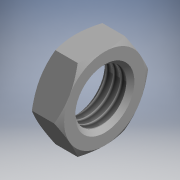
# Autodesk Inventor part: SNJ-010C
Saved by Autodesk Inventor 2017.3 (Build 213256000, 256)
## iProperties
Part Number: SNJ-010C
Material: Generic
Catalog Web Link: www.cadenas.de
Description: CJ2-Z_SNJ-Mounting Nut
Vendor: SMC
Document SubType Name: Modeling
Designer: partserver
Manufacturer: SMC
Mass: 0.259253 g
Surface Area: 3.5092 cm^2
Volume: 0.259253 cm^3
Density: 1 g/cm^3
Appearance: PSOLRGB-191-191-191
Category: PARTsolutions
Company: SMC
Title: SNJ-010C
Author: Cadenas PARTsolutions
Comments: Mounting Nut
PSOL_IDENT_0: {$CADENAS_DATA\23d-libs\smc_jp\actuator\standard_air_cylinder\cj2\accessories\cj2_z_snj.prj},159 {VT
PSOL_IDENT_1: YP=3D},{NB=SNJ-010C},{LINA=SNJ-010C},{NN=CJ2-Z_SNJ},{DATE=04.02.2022 06:57:30},{GEOMDATE=12.05.2020
PSOL_IDENT_2: 08:15:39},{VERSION=},{LINEID=90},{WBVAR=},{WBNUMERIC=}  {NB=SNJ-010C},{LINA=SNJ-010C},{KT=DUMMY},{MO
PSOL_IDENT_3: DEL=SNJ-010C},{BORE=10},{B1=11},{C1=12.7},{D=M8x1.0},{D1=8},{D2=1},{H1=4},{ORDER=SNJ-010C}
NB: SNJ-010C
NN: CJ2-Z_SNJ
NT: Mounting Nut
NBSYN: $MODEL.
LINA: SNJ-010C
CATALOG: SMC (JP
MODEL: SNJ-010C
BORE: 10
B1: 11
C1: 12.7
D: M8x1.0
H1: 4
SUPPLIER: SMC
ARTICLENO: SNJ-010C
BOMINFO: SNJ-010C
CREATOR: CADENAS GmbH
Autodesk Inventor part; units mm, degrees
sketch "B" plane through (0, 0, 0) normal (1, 0, 0) x (0, 1, 0)
  line L0 (-3.1754, 5.5) -> (-6.3509, 0)
  line L1 (-6.3509, 0) -> (-3.1754, -5.5)
  line L2 (-3.1754, -5.5) -> (3.1754, -5.5)
  line L3 (3.1754, -5.5) -> (6.3509, 0)
  line L4 (6.3509, 0) -> (3.1754, 5.5)
  line L5 (3.1754, 5.5) -> (-3.1754, 5.5)
  constraints: 12 end point
extrude "Extrusion1" add sketch "B" along normal mid plane 4
sketch "Sketch_2" plane through (0, 0, 0) normal (0, 0, 1) x (1, 0, 0)
  line L0 (2, 0) -> (-2, 0)
  line L1 (-2, 0) -> (-2, 4)
  line L2 (-2, 4) -> (-1.4585, 3.4585)
  line L3 (-1.4585, 3.4585) -> (1.4585, 3.4585)
  line L4 (1.4585, 3.4585) -> (2, 4)
  line L5 (2, 4) -> (2, 0)
  line L6 (2, 0) -> (-2, 0)
  constraints: 14 end point
revolve "Revolution1" cut sketch "Sketch_2" angle 360 about axis through (2, 0, 0) along (1, 0, 0)
thread "Thread1" size "M8x1" class "6H" standard "ISO Metric profile" full length
sketch "Sketch_3" plane through (0, 0, 0) normal (0, 0, 1) x (1, 0, 0)
  line L0 (50, 0) -> (-50, 0)
  line L1 (-7, 1) -> (-2, 1)
  line L2 (-2, 1) -> (-2, 5.5)
  line L3 (-2, 5.5) -> (0, 8.9641)
  line L4 (0, 8.9641) -> (2, 5.5)
  line L5 (2, 5.5) -> (2, 1)
  line L6 (2, 1) -> (7, 1)
  line L7 (7, 1) -> (7, 13.5)
  line L8 (7, 13.5) -> (-7, 13.5)
  line L9 (-7, 13.5) -> (-7, 1)
  constraints: 20 end point
revolve "Revolution2" cut sketch "Sketch_3" angle 360 about axis through (50, 0, 0) along (1, 0, 0)
ref_plane "nt_XY" through (0, 0, 0) normal (1, 0, 0) x (0, 0, -1)
ref_plane "nt_YZ" through (0, 0, 0) normal (0, 0, -1) x (0, 1, 0)
ref_plane "nt_ZX" through (0, 0, 0) normal (0, 1, 0) x (1, 0, 0)
ref_plane "ntj_XY" through (2, 0, 0) normal (1, 0, 0) x (0, 0, -1)
ref_plane "ntj_YZ" through (2, 0, 0) normal (0, 0, -1) x (0, 1, 0)
ref_plane "ntj_ZX" through (2, 0, 0) normal (0, 1, 0) x (1, 0, 0)
body "Solid1"
